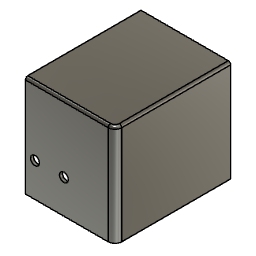
오른쪽 뒷 범퍼 (Autodesk Fusion 360 design; units mm, degrees)
Autodesk Fusion 360 part; units mm, degrees
sketch "스케치1" plane through (0, 0, 0) normal (0, 1, 0) x (1, 0, 0)
  line L0 (0, 0) -> (0, -105)
  line L1 (0, -105) -> (-93, -105)
  line L2 (-93, -105) -> (-93, -100)
  line L3 (-93, -100) -> (-6, -100)
  line L4 (-6, -100) -> (-6, 0)
  line L5 (-6, 0) -> (0, 0)
  line L6 (-93, -100) -> (-93, -102)
  line L7 (-93, -102) -> (-3, -102)
  line L8 (-3, -102) -> (-3, 0)
  dimension "d1" = 105
  dimension "d2" = 93
  dimension "d3" = 5
  dimension "d4" = 87
  dimension "d5" = 2
  dimension "d6" = 90
  constraint coincident L0.start L5.end
  constraint vertical L0
  constraint perpendicular L0 L1
  constraint perpendicular L1 L2
  constraint perpendicular L0 L3
  constraint perpendicular L3 L4
  constraint perpendicular L0 L5
  constraint coincident L2 L6.end
  constraint perpendicular L0 L7
  constraint midpoint L5 L8.end
  measures "d1" distance of L0.start L0.end
  measures "d2" distance of L0.end L1.end
  measures "d3" distance of L1.end L2.end
  measures "d4" distance of L2.end L3.end
  measures "d5" distance of L2.end L6.end
  measures "d6" distance of L6.end L7.end
extrude "돌출1" add sketch "스케치1" against normal blind 120 contours L0 L1 L2 L5 L7 L8
extrude "돌출2" add sketch "스케치1" against normal blind 3 contours L2 L3 L4 L5 L6 L7 L8
sketch "스케치2" plane through (-3, 0, 0) normal (-1, 0, 0) x (0, -1, 0)
  line L0 (3, 102) -> (3, 0)
  line L1 (3, 0) -> (120, 0)
  line L2 (120, 0) -> (120, 102)
  line L3 (120, 102) -> (3, 102)
  line L4 (120, 0) -> (117, 0)
  line L5 (117, 0) -> (117, 102)
  line L6 (117, 102) -> (120, 102)
  line L7 (120, 102) -> (120, 0)
  dimension "d11" = 3
  constraint horizontal L4
  constraint vertical L5
  constraint horizontal L6
  constraint vertical L7
  constraint coincident L1.end L2.start
  measures "d11" distance of L1.end L4.end
extrude "돌출3" add sketch "스케치2" along normal blind 90 contours L1 L2 L3 L4 L5 L6 L7
sketch "스케치3" plane through (-3, 0, 0) normal (-1, 0, 0) x (0, -1, 0)
  line L0 (117, 0) -> (117, 102)
  line L1 (117, 102) -> (3, 102)
  line L2 (3, 102) -> (3, 0)
  line L3 (3, 0) -> (117, 0)
  line L4 (117, 0) -> (116, 0)
  line L5 (116, 0) -> (8, 0)
  line L6 (8, 0) -> (8, 100)
  line L7 (8, 100) -> (116, 100)
  line L8 (116, 100) -> (116, 0)
  line L9 (8, 100) -> (29, 100)
  line L10 (29, 100) -> (29, 73.5)
  line L11 (29, 73.5) -> (8, 73.5)
  line L12 (8, 73.5) -> (8, 100)
  line L13 (33.5, 78) -> (24.5, 78)
  line L14 (24.5, 78) -> (24.5, 69)
  line L15 (24.5, 69) -> (33.5, 69)
  line L16 (33.5, 69) -> (33.5, 78)
  line L17 (33.5, 78) -> (24.5, 69) construction
  line L18 (24.5, 78) -> (33.5, 69) construction
  line L19 (116, 100) -> (113, 100)
  line L20 (116, 97) -> (116, 100)
  line L21 (8, 0) -> (12, 0)
  line L22 (12, 0) -> (12, 20)
  line L23 (12, 20) -> (8, 20)
  line L24 (8, 20) -> (8, 0)
  line L25 (15, 23) -> (9, 23)
  line L26 (9, 23) -> (9, 17)
  line L27 (9, 17) -> (15, 17)
  line L28 (15, 17) -> (15, 23)
  line L29 (15, 23) -> (9, 17) construction
  line L30 (9, 23) -> (15, 17) construction
  line L31 (116, 0) -> (107, 0)
  line L32 (107, 0) -> (107, 8)
  line L33 (107, 8) -> (116, 8)
  line L34 (116, 8) -> (116, 0)
  line L35 (102, 13) -> (112, 13)
  line L36 (112, 13) -> (112, 3)
  line L37 (112, 3) -> (102, 3)
  line L38 (102, 3) -> (102, 13)
  line L39 (102, 13) -> (112, 3) construction
  line L40 (112, 13) -> (102, 3) construction
  circle A0 centre (12, 20) radius 1.6
  circle A1 centre (29, 73.5) radius 2.1
  circle A2 centre (107, 8) radius 2.1
  line L41 (107, 8) -> (107, 75)
  line L42 (107, 75) -> (113, 75)
  circle A3 centre (113, 75) radius 1.6
  line L43 (110, 78) -> (116, 78)
  line L44 (116, 78) -> (116, 72)
  line L45 (116, 72) -> (110, 72)
  line L46 (110, 72) -> (110, 78)
  line L47 (110, 78) -> (116, 72) construction
  line L48 (116, 78) -> (110, 72) construction
  line L49 (112, 13) -> (117, 13)
  line L50 (117, 13) -> (117, 3)
  line L51 (117, 3) -> (112, 3)
  line L52 (112, 3) -> (112, 13)
  line L53 (116, 78) -> (117, 78)
  line L54 (117, 78) -> (117, 72)
  line L55 (117, 72) -> (116, 72)
  line L56 (116, 72) -> (116, 78)
  point P0 (29, 73.5)
  point P1 (12, 20)
  point P2 (107, 8)
  point P3 (113, 75)
  dimension "d14" = 1
  dimension "d15" = 108
  dimension "d16" = 100
  dimension "d17" = 21
  dimension "d18" = 26.5
  dimension "d19" = 9
  dimension "d20" = 9
  dimension "d21" = 3
  dimension "d22" = 3
  dimension "d25" = 4
  dimension "d26" = 20
  dimension "d27" = 6
  dimension "d28" = 6
  dimension "d29" = 9
  dimension "d30" = 8
  dimension "d31" = 10
  dimension "d32" = 10
  dimension "d33" = 3.2
  dimension "d34" = 4.2
  dimension "d35" = 4.2
  dimension "d81" = 67
  dimension "d82" = 6
  dimension "d83" = 3.2
  dimension "d84" = 6
  dimension "d85" = 6
  constraint coincident L0.start L3.end
  constraint horizontal L4
  constraint horizontal L5
  constraint vertical L6
  constraint horizontal L7
  constraint vertical L8
  constraint horizontal L9
  constraint vertical L10
  constraint horizontal L11
  constraint vertical L12
  constraint horizontal L13
  constraint perpendicular L13 L14
  constraint parallel L13 L15
  constraint parallel L14 L16
  constraint coincident L17 P0
  constraint coincident L18 P0
  constraint coincident P0 L10.end
  constraint horizontal L19
  constraint vertical L20
  constraint horizontal L21
  constraint vertical L22
  constraint horizontal L23
  constraint vertical L24
  constraint horizontal L25
  constraint perpendicular L25 L26
  constraint parallel L25 L27
  constraint parallel L26 L28
  constraint coincident L29 P1
  constraint coincident L30 P1
  constraint coincident P1 L22.end
  constraint horizontal L31
  constraint vertical L32
  constraint horizontal L33
  constraint vertical L34
  constraint horizontal L35
  constraint perpendicular L35 L36
  constraint parallel L35 L37
  constraint parallel L36 L38
  constraint coincident L39 P2
  constraint coincident L40 P2
  constraint coincident P2 L32.end
  constraint parallel L32 L41
  constraint perpendicular L41 L42
  constraint coincident P3 L42.end
  constraint horizontal L43
  constraint perpendicular L43 L44
  constraint parallel L43 L45
  constraint parallel L44 L46
  constraint coincident L47 P3
  constraint coincident L48 P3
  constraint horizontal L49
  constraint vertical L50
  constraint horizontal L51
  constraint vertical L52
  constraint coincident L0 L50.end
  constraint horizontal L53
  constraint vertical L54
  constraint horizontal L55
  constraint vertical L56
  constraint coincident L0 L54.end
  measures "d14" distance of L0.start L4.end
  measures "d15" distance of L4.end L5.end
  measures "d16" distance of L4.end L7.end
  measures "d17" distance of L6.end L9.end
  measures "d18" distance of L6.end L11.end
  measures "d19" distance of L14.end L15.end
  measures "d20" distance of L13.end L14.end
  measures "d21" distance of L7.end L19.end
  measures "d22" distance of L7.end L20.start
  measures "d25" distance of L5.end L21.end
  measures "d26" distance of L5.end L23.end
  measures "d27" distance of L26.end L27.end
  measures "d28" distance of L25.end L26.end
  measures "d29" distance of L4.end L31.end
  measures "d30" distance of L4.end L33.end
  measures "d31" distance of L36.end L37.end
  measures "d32" distance of L35.end L36.end
  measures "d33" diameter of A0
  measures "d34" diameter of A1
  measures "d35" diameter of A2
  measures "d81" distance of P2 L41.end
  measures "d82" distance of L41.end P3
  measures "d83" diameter of A3
  measures "d84" distance of L44.end L45.end
  measures "d85" distance of L43.end L44.end
extrude "돌출4" add sketch "스케치3" along normal blind 6 contours L0 L8 L34 L49 L50 L51 | L8 L33 L34 L36 L51 L52 | L0 L8 L44 L53 L54 L55 L56 | L8 L33 L36 L49 L52 | L32 L33 L36 L37 A2 L52 | L32 L35 L37 L38 A2 L41 | L8 L43 L44 L45 L46 L56 | L33 L35 L36 A2 L41 L52 | L22 L23 L26 L27 A0 | L22 L23 L25 L26 L27 L28 A0 | L10 L11 L13 L14 A1 | L10 L11 L13 L14 L15 L16 A1
thread "나사산2" "ISO Metric profile 4.0 M4x0.7 6H" major diameter 4.1095 minor diameter 3.332 pitch 0.7 angle 60 modelled right hand crest width 0.193 on face at (-5, -27.3913, 74.8499) crest through (-3.175, -30.666, 73.5) on face at (-7, -107.0524, 10.0993) crest through (-3.175, -108.666, 8)
sketch "스케치4" plane through (-6, 0, 0) normal (-1, 0, 0) x (0, -1, 0)
  line L0 (0, 100) -> (0, 0)
  line L1 (0, 0) -> (3, 0)
  line L2 (3, 0) -> (3, 100)
  line L3 (3, 100) -> (0, 100)
  line L4 (3, 0) -> (0, 0)
  line L5 (0, 0) -> (0, 43)
  line L6 (0, 43) -> (3, 43)
  line L7 (3, 43) -> (3, 0)
  dimension "d43" = 43
  constraint horizontal L4
  constraint vertical L5
  constraint horizontal L6
  constraint vertical L7
  constraint coincident L1.end L2.start
  measures "d43" distance of L1.end L6.end
extrude "돌출5" add sketch "스케치4" along normal blind 10 contours L0 L1 L2 L4 L5 L6 L7
sketch "스케치5" plane through (0, 0, 0) normal (0, 1, 0) x (-1, 0, 0)
  line L0 (93, 100) -> (93, 105)
  line L1 (93, 105) -> (0, 105)
  line L2 (0, 105) -> (0, 0)
  line L3 (0, 0) -> (16, 0)
  line L4 (16, 0) -> (16, 43)
  line L5 (16, 43) -> (6, 43)
  line L6 (6, 43) -> (6, 100)
  line L7 (6, 100) -> (93, 100)
  line L8 (16, 43) -> (6, 43)
  line L9 (6, 43) -> (6, 0)
  line L10 (6, 0) -> (16, 0)
  line L11 (16, 0) -> (16, 43)
  line L12 (11, 0) -> (11, 11.5)
  line L13 (11, 11.5) -> (11, 31.5)
  circle A0 centre (11, 31.5) radius 2.15
  circle A1 centre (11, 11.5) radius 2.15
  dimension "d46" = 10
  dimension "d47" = 11.5
  dimension "d48" = 20
  dimension "d49" = 4.3
  dimension "d50" = 4.3
  constraint horizontal L8
  constraint vertical L9
  constraint horizontal L10
  constraint vertical L11
  constraint coincident L3 L9.end
  constraint coincident L4.end L5.start
  constraint midpoint L10 L12.start
  constraint perpendicular L3 L12
  constraint perpendicular L3 L13
  constraint coincident L13.end A0.centre
  constraint coincident L12.end L13.start
  measures "d46" distance of L4.end L5.end
  measures "d47" distance of L12.start L12.end
  measures "d48" distance of L12.end L13.end
  measures "d49" diameter of A0
  measures "d50" diameter of A1
extrude "돌출6" cut sketch "스케치5" against normal blind 3 contours L12 L13 A1 | L12 L13 A1 | A0
sketch "스케치6" plane through (-93, 0, 0) normal (-1, 0, 0) x (0, -1, 0)
  line L0 (0, 105) -> (0, 100)
  line L1 (0, 100) -> (3, 100)
  line L2 (3, 100) -> (3, 102)
  line L3 (3, 102) -> (117, 102)
  line L4 (117, 102) -> (117, 0)
  line L5 (117, 0) -> (120, 0)
  line L6 (120, 0) -> (120, 105)
  line L7 (120, 105) -> (0, 105)
  line L8 (117, 102) -> (117, 73)
  line L9 (3, 73) -> (3, 53)
  line L10 (3, 53) -> (117, 53)
  line L11 (117, 53) -> (117, 73)
  line L12 (3, 73) -> (23, 73)
  line L13 (23, 73) -> (23, 102)
  line L14 (23, 102) -> (3, 102)
  line L15 (3, 102) -> (3, 73)
  line L16 (23, 73) -> (3, 73)
  line L17 (3, 73) -> (3, 53)
  line L18 (3, 53) -> (23, 53)
  line L19 (23, 53) -> (23, 73)
  line L20 (117, 73) -> (97, 73)
  line L21 (97, 73) -> (77, 73)
  line L22 (77, 73) -> (77, 53)
  line L23 (77, 53) -> (97, 53)
  line L24 (97, 53) -> (97, 73)
  line L25 (23, 63) -> (77, 63)
  line L26 (23, 63) -> (13, 63)
  line L27 (13, 63) -> (13, 73)
  line L28 (13, 73) -> (23, 73)
  line L29 (23, 73) -> (23, 63)
  circle A0 centre (13, 63) radius 2.65
  circle A1 centre (87, 63) radius 2.65
  circle A2 centre (107, 63) radius 2.15
  dimension "d53" = 29
  dimension "d54" = 20
  dimension "d55" = 20
  dimension "d57" = 20
  dimension "d58" = 20
  dimension "d64" = 10
  dimension "d65" = 5.3
  dimension "d66" = 5.3
  dimension "d73" = 4.3
  constraint coincident L3.end L4.start
  constraint perpendicular L3 L8
  constraint vertical L9
  constraint horizontal L10
  constraint vertical L11
  constraint horizontal L12
  constraint vertical L13
  constraint horizontal L14
  constraint vertical L15
  constraint horizontal L16
  constraint vertical L17
  constraint horizontal L18
  constraint vertical L19
  constraint perpendicular L8 L20
  constraint horizontal L21
  constraint vertical L22
  constraint horizontal L23
  constraint vertical L24
  constraint coincident L10 L22.end
  constraint midpoint L19 L25.start
  constraint midpoint L22 L25.end
  constraint horizontal L26
  constraint vertical L27
  constraint horizontal L28
  constraint vertical L29
  constraint coincident L26.end L27.start
  measures "d53" distance of L3.end L8.end
  measures "d54" distance of L8.end L10.end
  measures "d55" distance of L9.start L12.end
  measures "d57" distance of L8.end L20.end
  measures "d58" distance of L20.end L21.end
  measures "d64" distance of L25.start L26.end
  measures "d65" diameter of A0
  measures "d66" diameter of A1
  measures "d73" diameter of A2
extrude "돌출7" add sketch "스케치6" against normal blind 5 contours L2 L3 L12 L13 L14 L15 L16 L28 | L9 L10 L12 L16 L17 L18 L19 L26 L27 A0 | L12 L16 L19 L26 L27 L28 L29 A0 | L4 L10 L11 L20 L24 | L10 L19 L22 L25 | L10 L21 L22 L23 L24
extrude "돌출8" add 1 faces at (-89.6667, -3, 84.3333) along direction (0, 1, 0) blind 3
fillet "필렛1" radius 2.5 2 edges at (0, -60, 105) (-46.5, -120, 105)
fillet "필렛2" radius 7 2 edges at (0, -120, 51.25) (-0.7322, -119.2678, 104.2678)
sketch "스케치7" plane through (0, -117, 0) normal (0, 1, 0) x (-1, 0, 0)
  line L0 (88, 73) -> (93, 73)
  line L1 (93, 73) -> (93, 102)
  line L2 (93, 102) -> (3, 102)
  line L3 (3, 0) -> (93, 0)
  line L4 (93, 0) -> (93, 53)
  line L5 (93, 53) -> (88, 53)
  line L6 (88, 53) -> (88, 73)
  line L7 (3, 102) -> (3, 78)
  line L8 (3, 78) -> (9, 78)
  line L9 (9, 78) -> (9, 72)
  line L10 (9, 72) -> (3, 72)
  line L11 (3, 72) -> (3, 13)
  line L12 (3, 13) -> (9, 13)
  line L13 (9, 13) -> (9, 3)
  line L14 (9, 3) -> (3, 3)
  line L15 (3, 3) -> (3, 0)
  line L16 (93, 0) -> (83, 0)
  line L17 (83, 0) -> (83, 35)
  line L18 (83, 35) -> (93, 35)
  line L19 (93, 35) -> (93, 0)
  circle A0 centre (83, 35) radius 4.6
  line L20 (83, 35) -> (53, 35)
  circle A1 centre (53, 35) radius 4.6
  dimension "d86" = 10
  dimension "d87" = 35
  dimension "d88" = 9.2
  dimension "d89" = 30
  dimension "d90" = 9.2
  constraint horizontal L16
  constraint vertical L17
  constraint horizontal L18
  constraint vertical L19
  constraint coincident L3.end L4.start
  constraint coincident L17.end L18.start
  constraint perpendicular L17 L20
  constraint coincident L20.end A1.centre
  measures "d86" distance of L3.end L16.end
  measures "d87" distance of L3.end L18.end
  measures "d88" diameter of A0
  measures "d89" distance of L17.end L20.end
  measures "d90" diameter of A1
extrude "돌출9" cut sketch "스케치7" against normal blind 95 contours L17 L18 A0 | L18 A0 L20 | L17 A0 L20 | A1
thread "나사산3" "ISO Metric profile 3.0 M3x0.5 6H" major diameter 3.086 minor diameter 2.529 pitch 0.5 angle 60 modelled right hand crest width 0.1368 on face at (-7, -13.592, 19.8407) crest through (-3.125, -13.2645, 20) on face at (-7, -113.0399, 76.5995) crest through (-3.125, -114.2645, 75)
